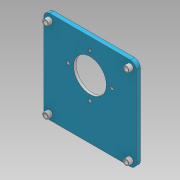
# Autodesk Inventor part: 연결부
Saved by Autodesk Inventor 2018 (Build 220112000, 112)
## iProperties
Created: 2018-04-05
Part Number: 연결부
Material: 일반
Document SubType Name: Modeling
Designer: CK
Density: 1 g/cm^3
Appearance: 기본값
Mass: 51.2428 g
Surface Area: 256.646 cm^2
Volume: 51.2428 cm^3
Author: CK
Autodesk Inventor part; units mm, degrees
ref_plane "YZ Plane" through (0, 0, 0) normal (1, 0, 0) x (0, 1, 0)
ref_plane "XZ Plane" through (0, 0, 0) normal (0, 1, 0) x (-1, 0, 0)
ref_plane "XY Plane" through (0, 0, 0) normal (0, 0, 1) x (1, 0, 0)
sketch "스케치1" plane through (0, 0, 0) normal (0, 1, 0) x (-1, 0, 0)
  line L0 (-55, 55) -> (55, 55)
  line L1 (55, 55) -> (55, -55)
  line L2 (55, -55) -> (-55, -55)
  line L3 (-55, -55) -> (-55, 55)
  line L4 (-55, 55) -> (55, -55) construction
  line L5 (55, 55) -> (-55, -55) construction
  point P0 (0, 0)
  dimension "d0" = 110
  dimension "d1" = 110
  constraints: 12 end point, 2 midpoint, 2 parallel, 1 horizontal, 1 perpendicular
  measures "d0" distance of L1.end L2.end
  measures "d1" distance of L0.end L1.end
extrude "돌출1" add sketch "스케치1" along normal blind 5
fillet "모깎기1" radius 7 1 edges at (55, 2.5, 55)
fillet "모깎기2" radius 7 3 edges at (55, 2.5, -55) (-55, 2.5, -55) (-55, 2.5, 55)
sketch "스케치9" plane through (0, 5, 0) normal (0, 1, 0) x (1, 0, 0)
  circle A0 centre (0, -15) radius 32.5
  line L0 (42.9638, 0) -> (-42.9638, 0) construction
  point P0 (0, 0)
  dimension "d32" = 65
  dimension "d33" = 15
  constraints: 2 end point, 1 centre point, 1 horizontal
  measures "d32" diameter of A0
  measures "d33" distance from line of L0 A0.centre
extrude "돌출9" cut sketch "스케치9" against normal blind 1
sketch "스케치10" plane through (0, 4, 15) normal (0, 1, 0) x (1, 0, 0)
  circle A0 centre (0, 0) radius 22.5
  point P0 (0, 15)
  dimension "d36" = 45
  constraints: 1 centre point
  measures "d36" diameter of A0
extrude "돌출10" cut sketch "스케치10" against normal blind 1
sketch "스케치11" plane through (0, 3, 15) normal (0, 1, 0) x (1, 0, 0)
  circle A0 centre (0, 0) radius 19.5
  point P0 (0, 15)
  dimension "d39" = 39
  constraints: 1 centre point
  measures "d39" diameter of A0
extrude "돌출11" cut sketch "스케치11" against normal through all
chamfer "모따기2" distance 1 angle 45 1 edges at (-22.5, 4, 15)
sketch "스케치12" plane through (0, 4, 15) normal (0, 1, 0) x (1, 0, 0)
  circle A0 centre (0, 0) radius 26 construction
  circle A1 centre (0, -26) radius 2
  point P0 (0, 15)
  dimension "d48" = 52
  dimension "d49" = 4
  constraints: 1 centre point, 1 vertical alignment, 2 other
  measures "d49" diameter of A1
extrude "돌출12" cut sketch "스케치12" against normal blind 10
pattern_circular "원형 패턴1" count 4 over 360 about axis through (0, 3.5, 15) along (0, 1, 0) of "돌출12"
sketch "스케치15" plane through (0, 5, 0) normal (0, 1, 0) x (1, 0, 0)
  arc A0 (48, -55) -> (55, -48) centre (48, -48) ccw projected
  circle A1 centre (48, -48) radius 2.538
  circle A2 centre (48, -48) radius 2.5
  point P0 (0, 0)
  dimension "d58" = 5
  constraints: 2 centre point, 2 coincident
  measures "d58" diameter of A2
sketch "스케치16" plane through (0, 0, 0) normal (0, -1, 0) x (1, 0, 0)
  circle A0 centre (48, 48) radius 3.5
  point P0 (0, 0)
  dimension "d55" = 7
  constraints: 1 centre point, 1 coincident
  measures "d55" diameter of A0
extrude "돌출13" add sketch "스케치16" along normal blind 5
mirror "미러7" about plane through (0, 0, 0) normal (0, 0, 1) of "돌출13"
mirror "미러8" about plane through (0, 0, 0) normal (1, 0, 0) of "돌출13", "미러7"
extrude "돌출14" cut sketch "스케치15" against normal through all contours A2
mirror "미러9" about plane through (0, 0, 0) normal (0, 0, 1) of "돌출14"
mirror "미러10" about plane through (0, 0, 0) normal (1, 0, 0) of "돌출14", "미러9"
